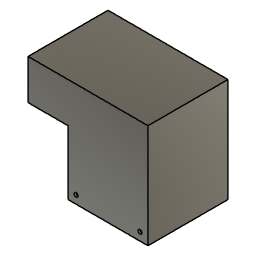
Piesa5_Proiect_PM (Autodesk Fusion 360 design; units mm, degrees)
Autodesk Fusion 360 part; units mm, degrees
note: some values were not read from the file. Set by a fixed rule: which face or edge a step refers to.
sketch "Sketch1" plane through (0, 0, 0) normal (0, 0, 1) x (1, 0, 0)
  line L0 (0, 0) -> (-100, 0)
  line L1 (-100, 0) -> (-100, 100)
  line L2 (-100, 100) -> (0, 100)
  line L3 (0, 100) -> (0, 0)
  dimension "d1" = 100
  dimension "d2" = 100
  constraint horizontal L0
  constraint vertical L1
  constraint horizontal L2
  constraint vertical L3
  constraint coincident L0.start L3.end
  measures "d1" distance of L0.start L0.end
  measures "d2" distance of L0.start L2.end
extrude "Extrude1" add sketch "Sketch1" along normal blind 50
shell "Shell1" thickness 5 removed faces 1 at (-33.3333, 33.3333, 0)
extrude "Extrude2" cut 1 faces at (-35, 35, 45) along direction (0, 0, 1) blind 55
sketch "Sketch2" plane through (0, 0, 0) normal (0, 0, -1) x (1, 0, 0)
  line L0 (-5, -5) -> (-5, -95)
  line L1 (-5, -95) -> (-95, -95)
  line L2 (-95, -95) -> (-95, -5)
  line L3 (-95, -5) -> (-5, -5)
  line L4 (-100, -100) -> (0, -100)
  line L5 (0, -100) -> (0, 0)
  line L6 (0, 0) -> (-100, 0)
  line L7 (-100, 0) -> (-100, -100)
  line L8 (-100, 0) -> (0, 0)
  line L9 (0, 0) -> (0, -100)
  line L10 (0, -100) -> (-100, -100)
  line L11 (-100, -100) -> (-100, 0)
  line L12 (-2.5, -97.5) -> (-97.5, -97.5)
  line L13 (-97.5, -97.5) -> (-97.5, -2.5)
  line L14 (-97.5, -2.5) -> (-2.5, -2.5)
  line L15 (-2.5, -2.5) -> (-2.5, -97.5)
  dimension "d8" = 2.5
  constraint horizontal L8
  constraint vertical L9
  constraint horizontal L10
  constraint vertical L11
  constraint coincident L4.end L5.start
  constraint coincident L6.end L7.start
extrude "Extrude3" add sketch "Sketch2" along normal blind 30 contours L4 L5 L6 L7 L8 L9 L10 L11
extrude "Extrude4" cut 1 faces at (-97.5, 65.8333, -10) along direction (-1, 0, 0) blind 40
sketch "Sketch3" plane through (0, 0, 0) normal (0, -1, 0) x (1, 0, 0)
  line L0 (0, -30) -> (0, 50)
  line L1 (0, 50) -> (-100, 50)
  line L2 (-100, 50) -> (-100, -30)
  line L3 (-100, -30) -> (0, -30)
  line L4 (-100, -30) -> (-90, -30)
  line L5 (-90, -30) -> (-90, -20)
  line L6 (-90, -20) -> (-100, -20)
  line L7 (-100, -20) -> (-100, -30)
  line L8 (0, -30) -> (-10, -30)
  line L9 (-10, -30) -> (-10, -20)
  line L10 (-10, -20) -> (0, -20)
  line L11 (0, -20) -> (0, -30)
  circle A0 centre (-90, -20) radius 2.5
  circle A1 centre (-10, -20) radius 2.5
  dimension "d13" = 5
  dimension "d14" = 5
  constraint horizontal L4
  constraint vertical L5
  constraint horizontal L6
  constraint vertical L7
  constraint coincident L2.end L3.start
  constraint horizontal L8
  constraint vertical L9
  constraint horizontal L10
  constraint vertical L11
  constraint coincident L0.start L3.end
  constraint coincident L5.end L6.start
  constraint coincident L9.end L10.start
  measures "d13" diameter of A0
  measures "d14" diameter of A1
extrude "Extrude5" cut sketch "Sketch3" against normal blind 160 contours L9 L10 A1 | L9 L10 A1 | L5 L6 A0 | L5 L6 A0
sketch "Sketch4" plane through (0, 0, 50) normal (0, 0, 1) x (-1, 0, 0)
  line L0 (5, -95) -> (5, -5)
  line L1 (5, -5) -> (95, -5)
  line L2 (95, -5) -> (95, -95)
  line L3 (95, -95) -> (5, -95)
  line L4 (0, -100) -> (100, -100)
  line L5 (100, -100) -> (100, 0)
  line L6 (100, 0) -> (0, 0)
  line L7 (0, 0) -> (0, -100)
  line L8 (0, 0) -> (150, 0)
  line L9 (150, 0) -> (150, -100)
  line L10 (150, -100) -> (0, -100)
  line L11 (0, -100) -> (0, 0)
  constraint horizontal L8
  constraint vertical L9
  constraint horizontal L10
  constraint vertical L11
  constraint coincident L6.end L7.start
extrude "Extrude6" add sketch "Sketch4" along normal blind 50
shell "Shell2" thickness 5 removed faces 1 at (-95, 35, 33.3333)
extrude "Extrude7" add 1 faces at (-95, 35, 96.6667) along direction (1, 0, 0) blind 90
sketch "Sketch5" plane through (-150, 0, 0) normal (-1, 0, 0) x (0, -1, 0)
  line L0 (-100, 50) -> (0, 50)
  line L1 (0, 50) -> (0, 100)
  line L2 (0, 100) -> (-100, 100)
  line L3 (-100, 100) -> (-100, 50)
  line L4 (-100, 50) -> (-85, 50)
  line L5 (-85, 50) -> (-85, 63.5)
  line L6 (-85, 63.5) -> (-100, 63.5)
  line L7 (-100, 63.5) -> (-100, 50)
  line L8 (-85, 63.5) -> (-15, 63.5)
  line L9 (-15, 63.5) -> (-15, 86.5)
  line L10 (-15, 86.5) -> (-85, 86.5)
  line L11 (-85, 86.5) -> (-85, 63.5)
  dimension "d22" = 15
  dimension "d23" = 13.5
  dimension "d24" = 70
  dimension "d25" = 23
  constraint horizontal L4
  constraint vertical L5
  constraint horizontal L6
  constraint vertical L7
  constraint coincident L0.start L3.end
  constraint horizontal L8
  constraint vertical L9
  constraint horizontal L10
  constraint vertical L11
  measures "d22" distance of L0.start L4.end
  measures "d23" distance of L0.start L6.end
  measures "d24" distance of L5.end L8.end
  measures "d25" distance of L5.end L10.end
extrude "Extrude8" cut sketch "Sketch5" against normal blind 40 contours L8 L9 L10 L11
sketch "Sketch6" plane through (-150, 0, 0) normal (-1, 0, 0) x (0, -1, 0)
  line L0 (-15, 63.5) -> (-85, 63.5)
  line L1 (-85, 63.5) -> (-85, 86.5)
  line L2 (-85, 86.5) -> (-15, 86.5)
  line L3 (-15, 86.5) -> (-15, 63.5)
  line L4 (-100, 50) -> (0, 50)
  line L5 (0, 50) -> (0, 100)
  line L6 (0, 100) -> (-100, 100)
  line L7 (-100, 100) -> (-100, 50)
  line L8 (-15, 86.5) -> (-12, 86.5)
  line L9 (-12, 86.5) -> (-12, 91.5)
  line L10 (-12, 91.5) -> (-15, 91.5)
  line L11 (-15, 91.5) -> (-15, 86.5)
  line L12 (-15, 63.5) -> (-12, 63.5)
  line L13 (-12, 63.5) -> (-12, 58.5)
  line L14 (-12, 58.5) -> (-15, 58.5)
  line L15 (-15, 58.5) -> (-15, 63.5)
  line L16 (-85, 86.5) -> (-88, 86.5)
  line L17 (-88, 86.5) -> (-88, 91.5)
  line L18 (-88, 91.5) -> (-85, 91.5)
  line L19 (-85, 91.5) -> (-85, 86.5)
  line L20 (-85, 63.5) -> (-88, 63.5)
  line L21 (-88, 63.5) -> (-88, 58.5)
  line L22 (-88, 58.5) -> (-85, 58.5)
  line L23 (-85, 58.5) -> (-85, 63.5)
  circle A0 centre (-88, 91.5) radius 2
  circle A1 centre (-12, 91.5) radius 2
  circle A2 centre (-88, 58.5) radius 2
  circle A3 centre (-12, 58.5) radius 2
  dimension "d28" = 3
  dimension "d29" = 5
  dimension "d30" = 5
  dimension "d31" = 3
  dimension "d32" = 5
  dimension "d33" = 5
  dimension "d34" = 4
  dimension "d35" = 4
  dimension "d36" = 4
  dimension "d37" = 4
  constraint horizontal L8
  constraint vertical L9
  constraint horizontal L10
  constraint vertical L11
  constraint coincident L2.end L3.start
  constraint horizontal L12
  constraint vertical L13
  constraint horizontal L14
  constraint vertical L15
  constraint coincident L0.start L3.end
  constraint horizontal L16
  constraint vertical L17
  constraint horizontal L18
  constraint vertical L19
  constraint coincident L1.end L2.start
  constraint horizontal L20
  constraint vertical L21
  constraint horizontal L22
  constraint vertical L23
  constraint coincident L0.end L1.start
  constraint coincident L17.end L18.start
  constraint coincident L9.end L10.start
  constraint coincident L21.end L22.start
  constraint coincident L13.end L14.start
  measures "d28" distance of L2.end L8.end
  measures "d29" distance of L2.end L10.end
  measures "d30" distance of L0.start L14.end
  measures "d31" distance of L1.end L16.end
  measures "d32" distance of L1.end L18.end
  measures "d33" distance of L0.end L22.end
  measures "d34" diameter of A0
  measures "d35" diameter of A1
  measures "d36" diameter of A2
  measures "d37" diameter of A3
extrude "Extrude9" cut sketch "Sketch6" against normal blind 10 contours L13 L14 A3 | L13 L14 A3 | L21 L22 A2 | L21 L22 A2 | L9 L10 A1 | L9 L10 A1 | L17 L18 A0 | L17 L18 A0
sketch "Sketch7" plane through (-150, 0, 0) normal (-1, 0, 0) x (0, -1, 0)
  circle A0 centre (-12, 91.5) radius 2
  circle A1 centre (-12, 58.5) radius 2
  circle A2 centre (-88, 91.5) radius 2
  circle A3 centre (-88, 58.5) radius 2
  line L0 (-15, 63.5) -> (-85, 63.5)
  line L1 (-85, 63.5) -> (-85, 86.5)
  line L2 (-85, 86.5) -> (-15, 86.5)
  line L3 (-15, 86.5) -> (-15, 63.5)
  line L4 (-100, 50) -> (0, 50)
  line L5 (0, 50) -> (0, 100)
  line L6 (0, 100) -> (-100, 100)
  line L7 (-100, 100) -> (-100, 50)
  line L8 (-85, 86.5) -> (-15, 86.5)
  line L9 (-15, 86.5) -> (-15, 63.5)
  line L10 (-15, 63.5) -> (-85, 63.5)
  line L11 (-85, 63.5) -> (-85, 86.5)
  line L12 (-13, 61.5) -> (-87, 61.5)
  line L13 (-87, 61.5) -> (-87, 88.5)
  line L14 (-87, 88.5) -> (-13, 88.5)
  line L15 (-13, 88.5) -> (-13, 61.5)
  dimension "d40" = -2
  constraint horizontal L8
  constraint vertical L9
  constraint horizontal L10
  constraint vertical L11
  constraint coincident L0.start L3.end
  constraint coincident L1.end L2.start
extrude "Extrude10" cut sketch "Sketch7" against normal blind 60 contours L12 L13 L14 L15
sketch "Sketch8" plane through (-150, 0, 0) normal (-1, 0, 0) x (0, -1, 0)
  line L0 (-87, 61.5) -> (-87, 88.5)
  line L1 (-87, 88.5) -> (-13, 88.5)
  line L2 (-13, 88.5) -> (-13, 61.5)
  line L3 (-13, 61.5) -> (-87, 61.5)
  circle A0 centre (-12, 91.5) radius 2
  circle A1 centre (-12, 58.5) radius 2
  circle A2 centre (-88, 91.5) radius 2
  circle A3 centre (-88, 58.5) radius 2
  line L4 (-100, 50) -> (0, 50)
  line L5 (0, 50) -> (0, 100)
  line L6 (0, 100) -> (-100, 100)
  line L7 (-100, 100) -> (-100, 50)
  circle A4 centre (-12, 91.5) radius 2.5
  circle A5 centre (-12, 58.5) radius 2.5
  circle A6 centre (-88, 91.5) radius 2.5
  circle A7 centre (-88, 58.5) radius 2.5
  dimension "d43" = 5
  dimension "d44" = 5
  dimension "d45" = 5
  dimension "d46" = 5
  constraint concentric A0 A4
  constraint concentric A1 A5
  constraint concentric A2 A6
  constraint concentric A3 A7
  measures "d43" diameter of A4
  measures "d44" diameter of A5
  measures "d45" diameter of A6
  measures "d46" diameter of A7
extrude "Extrude11" cut sketch "Sketch8" against normal blind 40 contours A4 | A5 | A6 | A7
